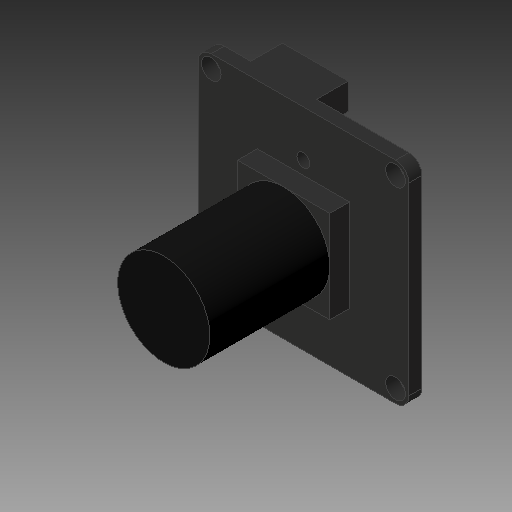
# Autodesk Inventor part: Camera
Saved by Autodesk Inventor 2019 (Build 230136000, 136)
## iProperties
Created: 2021-07-29
Part Number: Camera
Material: 일반
Document SubType Name: Modeling
Designer: user
Density: 1 g/cm^3
Appearance: 기본값
Mass: 5.55369 g
Surface Area: 34.2456 cm^2
Volume: 5.55369 cm^3
Author: user
Autodesk Inventor part; units mm, degrees
ref_plane "YZ Plane" through (0, 0, 0) normal (1, 0, 0) x (0, 1, 0)
ref_plane "XZ Plane" through (0, 0, 0) normal (0, 1, 0) x (-1, 0, 0)
ref_plane "XY Plane" through (0, 0, 0) normal (0, 0, 1) x (1, 0, 0)
sketch "스케치1" plane through (0, 0, 0) normal (0, 0, 1) x (1, 0, 0)
  line L0 (-16, 16) -> (16, 16)
  line L1 (16, 16) -> (16, -16)
  line L2 (16, -16) -> (-16, -16)
  line L3 (-16, -16) -> (-16, 16)
  point P0 (0, 0)
  dimension "d0" = 32
  dimension "d1" = 32
  dimension "d2" = 16
  dimension "d3" = 16
  constraints: 8 end point, 2 parallel, 1 horizontal, 1 perpendicular
  measures "d0" distance of L1.end L2.end
  measures "d1" distance of L0.end L1.end
  measures "d2" distance from line of point (0, 0) L0
  measures "d3" distance from line of L3 point (0, 0)
extrude "돌출1" add sketch "스케치1" along normal blind 2
sketch "스케치2" plane through (0, 0, 2) normal (0, 0, 1) x (1, 0, 0)
  circle A0 centre (-14, 14) radius 1.5
  circle A1 centre (14, 14) radius 1.5
  circle A2 centre (-14, -14) radius 1.5
  circle A3 centre (14, -14) radius 1.5
  line L0 (-16, 16) -> (-16, -16) projected
  line L1 (16, 16) -> (-16, 16) projected
  line L2 (-16, -16) -> (16, -16) projected
  line L3 (16, -16) -> (16, 16) projected
  point P0 (0, 0)
  dimension "d6" = 3
  dimension "d7" = 3
  dimension "d8" = 3
  dimension "d9" = 3
  dimension "d10" = 28
  dimension "d12" = 28
  dimension "d13" = 2
  dimension "d14" = 14
  dimension "d15" = 2
  dimension "d16" = 2
  dimension "d17" = 2
  dimension "d18" = 2
  dimension "d19" = 2
  dimension "d20" = 2
  constraints: 4 centre point
  measures "d6" diameter of A0
  measures "d7" diameter of A1
  measures "d8" diameter of A2
  measures "d9" diameter of A3
  measures "d10" distance of A2.centre A0.centre
  measures "d12" distance of A1.centre A0.centre
  measures "d13" distance from line of L0 A2.centre
  measures "d14" horizontal distance of A2.centre point (0, 0)
  measures "d15" distance from line of L0 A0.centre
  measures "d16" distance from line of L1 A1.centre
  measures "d17" distance from line of L2 A3.centre
  measures "d18" distance from line of L3 A3.centre
  measures "d19" distance from line of L1 A0.centre
  measures "d20" distance from line of L3 A1.centre
extrude "돌출2" cut sketch "스케치2" against normal up to surface (2 mm away) contours A0 | A1 | A2 | A3
sketch "스케치3" plane through (0, 0, 2) normal (0, 0, 1) x (1, 0, 0)
  line L0 (-7, 7) -> (7, 7)
  line L1 (7, 7) -> (7, -7)
  line L2 (7, -7) -> (-7, -7)
  line L3 (-7, -7) -> (-7, 7)
  point P0 (0, 0)
  dimension "d23" = 7
  dimension "d24" = 14
  dimension "d25" = 7
  dimension "d26" = 14
  constraints: 8 end point, 2 parallel, 1 horizontal, 1 perpendicular
  measures "d23" distance from line of point (0, 0) L3
  measures "d24" distance between parallel lines of L1 L3
  measures "d25" distance from line of point (0, 0) L2
  measures "d26" distance between parallel lines of L2 L0
extrude "돌출3" add sketch "스케치3" along normal blind 3
sketch "스케치4" plane through (0, 0, 5) normal (0, 0, 1) x (1, 0, 0)
  circle A0 centre (0, 0) radius 7
  dimension "d29" = 14
  constraints: 1 centre point, 1 coincident
  measures "d29" diameter of A0
extrude "돌출4" add sketch "스케치4" along normal blind 18.2
sketch "스케치6" plane through (0, 0, 2) normal (0, 0, 1) x (1, 0, 0)
  circle A0 centre (0, 9) radius 1
  circle A1 centre (0, -9) radius 1
  line L0 (7, 7) -> (0, 7) projected
  line L1 (0, -7) -> (7, -7) projected
  line L2 (-16, 16) -> (-16, -16) projected
  point P0 (0, 0)
  dimension "d32" = 2
  dimension "d33" = 2
  dimension "d34" = 2
  dimension "d35" = 2
  dimension "d36" = 16
  dimension "d37" = 16
  constraints: 2 centre point
  measures "d32" diameter of A0
  measures "d33" diameter of A1
  measures "d34" distance from line of L0 A0.centre
  measures "d35" distance from line of L1 A1.centre
  measures "d36" distance from line of L2 A1.centre
  measures "d37" distance from line of L2 A0.centre
extrude "돌출5" cut sketch "스케치6" against normal up to surface (2 mm away)
sketch "스케치5" plane through (0, 0, 0) normal (0, 0, -1) x (-1, 0, 0)
  line L0 (-16, 16) -> (16, 16) projected
  line L1 (10, 12) -> (0, 12)
  line L2 (0, 12) -> (0, 16)
  line L3 (0, 16) -> (10, 16)
  line L4 (10, 16) -> (10, 12)
  point P0 (0, 0)
  dimension "d40" = 4
  dimension "d41" = 10
  constraints: 8 end point, 2 parallel, 1 horizontal, 1 midpoint, 1 perpendicular
  measures "d40" distance between parallel lines of L0 L1
  measures "d41" distance between parallel lines of L2 L4
extrude "돌출6" add sketch "스케치5" along normal blind 4.8
fillet "모깎기1" radius 2 4 edges at (-16, -16, 1) (-16, 16, 1) (16, 16, 1) (16, -16, 1)
equation "\"d2\" = 0.5 * d1"
equation "\"d3\" = 0.5 * d0"
